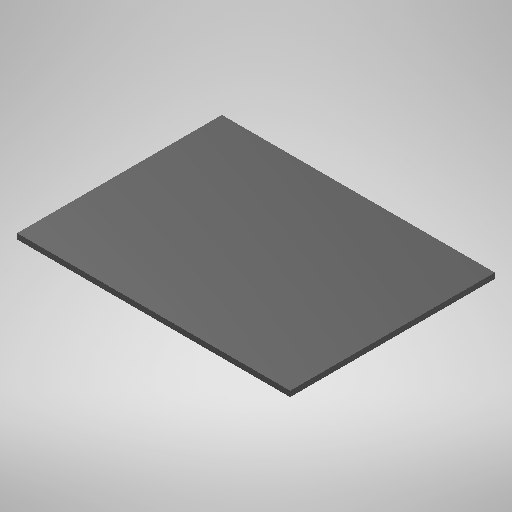
# Autodesk Inventor part: veraboard
Saved by Autodesk Inventor 2025.2 (Build 292293000, 293)
## iProperties
Created: 2025-08-16
Part Number: veraboard
Material: Copper
Document SubType Name: Modeling
Designer: pakiyan
Density: 8.94 g/cm^3
Appearance: Copper - Satin
Author: pakiyan
Autodesk Inventor part; units mm, degrees
ref_plane "YZ Plane" through (0, 0, 0) normal (1, 0, 0) x (0, 1, 0)
ref_plane "XZ Plane" through (0, 0, 0) normal (0, 1, 0) x (-1, 0, 0)
ref_plane "XY Plane" through (0, 0, 0) normal (0, 0, 1) x (1, 0, 0)
sketch "Sketch1" plane through (0, 0, 0) normal (0, 1, 0) x (-1, 0, 0)
  line L0 (50, 37.5) -> (-50, 37.5)
  line L1 (-50, 37.5) -> (-50, -37.5)
  line L2 (-50, -37.5) -> (50, -37.5)
  line L3 (50, -37.5) -> (50, 37.5)
  line L4 (50, 37.5) -> (-50, -37.5) construction
  line L5 (-50, 37.5) -> (50, -37.5) construction
  point P0 (0, 0)
  dimension "d0" = 100
  dimension "d1" = 75
  constraints: 12 end point, 2 midpoint, 2 parallel, 1 horizontal, 1 perpendicular
  measures "d0" distance of L0.start L0.end
  measures "d1" distance of L0.end L1.end
extrude "Extrusion1" add sketch "Sketch1" along normal blind 2
body "Solid1"
